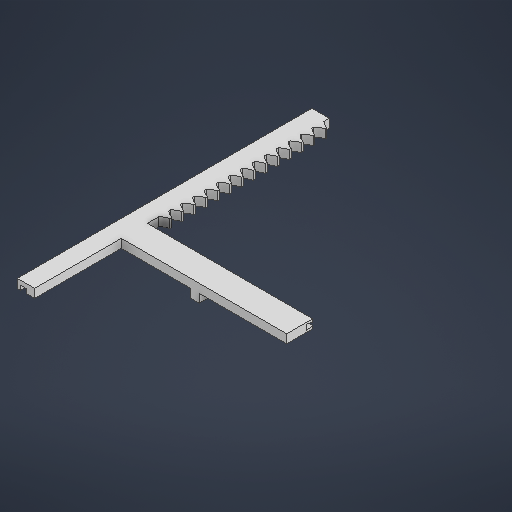
# Autodesk Inventor part: Rack
Saved by Autodesk Inventor 2026.1 (Build 301233020, 233B)
## iProperties
Created: 2025-10-17
Part Number: Rack
Material: Generic
Document SubType Name: Modeling
Designer: alexj
Density: 1 g/cm^3
Appearance: Default
Author: alexj
Autodesk Inventor part; units mm, degrees
ref_plane "YZ Plane" through (0, 0, 0) normal (1, 0, 0) x (0, 1, 0)
ref_plane "XZ Plane" through (0, 0, 0) normal (0, 1, 0) x (-1, 0, 0)
ref_plane "XY Plane" through (0, 0, 0) normal (0, 0, 1) x (1, 0, 0)
sketch "Sketch1" plane through (0, 0, 0) normal (0, 1, 0) x (-1, 0, 0)
  line L0 (0, 0) -> (10, 0)
  line L1 (10, 0) -> (10, -170)
  line L2 (10, -170) -> (0, -170)
  line L3 (0, -170) -> (0, 0)
  dimension "d0" = 170
  dimension "d1" = 10
  constraints: 8 end point, 2 parallel, 1 horizontal, 1 perpendicular
  measures "d0" distance of L0.end L1.end
  measures "d1" distance of L1.end L2.end
extrude "Extrusion1" add sketch "Sketch1" along normal blind 5
sketch "Sketch2" plane through (-10, 0, 0) normal (0, 0, 1) x (1, 0, 0)
  line L0 (2, 0) -> (2, 2.5)
  line L1 (2, 2.5) -> (5, 2.5)
  line L2 (0, 0) -> (0, 5) projected
  line L3 (5, 2.5) -> (5, 0)
  line L4 (0, 0) -> (10, 0) projected
  dimension "d6" = 2
  dimension "d9" = 3
  dimension "d75" = 2.5
  constraints: 6 end point, 1 midpoint, 1 perpendicular, 1 point on line, 1 vertical
  measures "d6" distance between parallel lines of L2 L0
  measures "d9" distance of L0.end L1.end
  measures "d75" distance between parallel lines of L4 L1
sketch "Sketch4" plane through (0, 5, 0) normal (0, 1, 0) x (1, 0, 0)
  line L0 (95.426, 50) -> (95.426, 65)
  line L1 (95.426, 65) -> (0, 65)
  line L2 (95.426, 50) -> (0, 50)
  line L3 (-10, 0) -> (0, 0) projected
  line L4 (0, 0) -> (0, 170) projected
  line L5 (0, 50) -> (0, 65)
  dimension "d107" = 95.426
  dimension "d108" = 15
  dimension "d109" = 50
  constraints: 9 end point, 2 perpendicular, 1 horizontal, 1 parallel, 1 point on line, 1 vertical
  measures "d107" distance from line of L3.end L0
  measures "d108" distance between parallel lines of L1 L2
  measures "d109" distance from line of L3.end L2
extrude "Extrusion4" add sketch "Sketch4" against normal blind 5
sketch "Sketch6" plane through (0, 5, 0) normal (0, 1, 0) x (1, 0, 0)
  line L0 (0, 0) -> (0, 170) projected
  line L1 (95.426, 50) -> (95.426, 65) projected
  arc A0 (4.0959, 156.5581) -> (0, 154.1943) centre (6.5788, 147.5251) ccw
  arc A1 (4.0959, 157.6362) -> (4.0959, 156.5581) centre (9.5694, 157.0972) ccw
  arc A2 (0, 160) -> (4.0959, 157.6362) centre (6.5788, 166.6692) ccw
  line L2 (0, 154.1943) -> (0, 160)
  arc A3 (4.0959, 163.4421) -> (0, 161.0783) centre (6.5788, 154.4091) ccw
  arc A4 (4.0959, 164.5202) -> (4.0959, 163.4421) centre (9.5694, 163.9812) ccw
  arc A5 (0, 166.884) -> (4.0959, 164.5202) centre (6.5788, 173.5532) ccw
  arc A6 (4.0959, 149.6741) -> (0, 147.3103) centre (6.5788, 140.6411) ccw
  arc A7 (4.0959, 150.7522) -> (4.0959, 149.6741) centre (9.5694, 150.2132) ccw
  arc A8 (0, 153.116) -> (4.0959, 150.7522) centre (6.5788, 159.7852) ccw
  arc A9 (4.0959, 142.7901) -> (0, 140.4263) centre (6.5788, 133.7571) ccw
  arc A10 (4.0959, 143.8682) -> (4.0959, 142.7901) centre (9.5694, 143.3292) ccw
  arc A11 (0, 146.232) -> (4.0959, 143.8682) centre (6.5788, 152.9012) ccw
  arc A12 (4.0959, 135.9061) -> (0, 133.5423) centre (6.5788, 126.8731) ccw
  arc A13 (4.0959, 136.9842) -> (4.0959, 135.9061) centre (9.5694, 136.4452) ccw
  arc A14 (0, 139.348) -> (4.0959, 136.9842) centre (6.5788, 146.0172) ccw
  arc A15 (4.0959, 129.0221) -> (0, 126.6583) centre (6.5788, 119.9891) ccw
  arc A16 (4.0959, 130.1002) -> (4.0959, 129.0221) centre (9.5694, 129.5612) ccw
  arc A17 (0, 132.464) -> (4.0959, 130.1002) centre (6.5788, 139.1332) ccw
  arc A18 (4.0959, 122.1381) -> (0, 119.7743) centre (6.5788, 113.1051) ccw
  arc A19 (4.0959, 123.2162) -> (4.0959, 122.1381) centre (9.5694, 122.6772) ccw
  arc A20 (0, 125.58) -> (4.0959, 123.2162) centre (6.5788, 132.2492) ccw
  arc A21 (4.0959, 115.2541) -> (0, 112.8903) centre (6.5788, 106.2211) ccw
  arc A22 (4.0959, 116.3322) -> (4.0959, 115.2541) centre (9.5694, 115.7932) ccw
  arc A23 (0, 118.696) -> (4.0959, 116.3322) centre (6.5788, 125.3652) ccw
  arc A24 (4.0959, 108.3701) -> (0, 106.0063) centre (6.5788, 99.3371) ccw
  arc A25 (4.0959, 109.4482) -> (4.0959, 108.3701) centre (9.5694, 108.9092) ccw
  arc A26 (0, 111.812) -> (4.0959, 109.4482) centre (6.5788, 118.4812) ccw
  arc A27 (4.0959, 101.4861) -> (0, 99.1223) centre (6.5788, 92.4531) ccw
  arc A28 (4.0959, 102.5642) -> (4.0959, 101.4861) centre (9.5694, 102.0252) ccw
  arc A29 (0, 104.928) -> (4.0959, 102.5642) centre (6.5788, 111.5972) ccw
  arc A30 (4.0959, 94.6021) -> (0, 92.2383) centre (6.5788, 85.5691) ccw
  arc A31 (4.0959, 95.6802) -> (4.0959, 94.6021) centre (9.5694, 95.1412) ccw
  arc A32 (0, 98.044) -> (4.0959, 95.6802) centre (6.5788, 104.7132) ccw
  arc A33 (4.0959, 87.7181) -> (0, 85.3543) centre (6.5788, 78.6851) ccw
  arc A34 (4.0959, 88.7962) -> (4.0959, 87.7181) centre (9.5694, 88.2572) ccw
  arc A35 (0, 91.16) -> (4.0959, 88.7962) centre (6.5788, 97.8292) ccw
  arc A36 (4.0959, 80.8341) -> (0, 78.4703) centre (6.5788, 71.8011) ccw
  arc A37 (4.0959, 81.9122) -> (4.0959, 80.8341) centre (9.5694, 81.3732) ccw
  arc A38 (0, 84.276) -> (4.0959, 81.9122) centre (6.5788, 90.9452) ccw
  arc A39 (4.0959, 73.9501) -> (0, 71.5863) centre (6.5788, 64.9171) ccw
  arc A40 (4.0959, 75.0282) -> (4.0959, 73.9501) centre (9.5694, 74.4892) ccw
  arc A41 (0, 77.392) -> (4.0959, 75.0282) centre (6.5788, 84.0612) ccw
  point P0 (0, 65)
  point P1 (0, 154.1943)
  point P2 (0, 166.884)
  point P3 (0, 161.0783)
  point P4 (0, 77.392)
  point P5 (0, 71.5863)
  point P6 (0, 84.276)
  point P7 (0, 78.4703)
  point P8 (0, 91.16)
  point P9 (0, 85.3543)
  point P10 (0, 98.044)
  point P11 (0, 92.2383)
  point P12 (0, 104.928)
  point P13 (0, 99.1223)
  point P14 (0, 111.812)
  point P15 (0, 106.0063)
  point P16 (0, 118.696)
  point P17 (0, 112.8903)
  point P18 (0, 125.58)
  point P19 (0, 119.7743)
  point P20 (0, 132.464)
  point P21 (0, 126.6583)
  point P22 (0, 139.348)
  point P23 (0, 133.5423)
  point P24 (0, 146.232)
  point P25 (0, 140.4263)
  point P26 (0, 153.116)
  point P27 (0, 147.3103)
  dimension "d80" = 6.884
  dimension "d88" = 6.884
  dimension "d200" = 5.5
  dimension "d201" = 9.368
  dimension "d202" = 95.426
  dimension "d203" = 95.426
  dimension "d204" = 85.8566
  dimension "d205" = 88.8472
  dimension "d206" = 88.8472
  dimension "d207" = 91.3301
  dimension "d208" = 91.3301
  dimension "d209" = 95.426
  dimension "d210" = 95.426
  dimension "d211" = 95.426
  dimension "d212" = 95.426
  dimension "d213" = 95.426
  dimension "d214" = 95.426
  dimension "d215" = 95.426
  dimension "d216" = 95.426
  dimension "d217" = 95.426
  dimension "d218" = 95.426
  dimension "d219" = 95.426
  dimension "d220" = 95.426
  dimension "d221" = 95.426
  dimension "d222" = 95.426
  dimension "d223" = 95.426
  dimension "d224" = 95.426
  dimension "d225" = 95.426
  dimension "d226" = 95.426
  dimension "d227" = 95.426
  dimension "d228" = 95.426
  dimension "d229" = 95.426
  dimension "d230" = 95.426
  dimension "d231" = 95.426
  dimension "d232" = 95.426
  dimension "d233" = 95.426
  dimension "d234" = 95.426
  dimension "d235" = 95.426
  dimension "d236" = 95.426
  dimension "d237" = 131.0291
  dimension "d238" = 139.594
  dimension "d239" = 135.4148
  dimension "d240" = 134.6518
  dimension "d241" = 130.6206
  dimension "d242" = 129.8867
  dimension "d243" = 126.0203
  dimension "d244" = 125.3186
  dimension "d245" = 121.6357
  dimension "d246" = 120.97
  dimension "d247" = 117.4912
  dimension "d248" = 116.8654
  dimension "d249" = 113.6128
  dimension "d250" = 113.0312
  dimension "d251" = 110.0288
  dimension "d252" = 109.496
  dimension "d253" = 106.7689
  dimension "d254" = 106.2896
  dimension "d255" = 103.8636
  dimension "d256" = 103.4426
  dimension "d257" = 101.3432
  dimension "d258" = 100.9853
  dimension "d259" = 99.2373
  dimension "d260" = 98.9468
  dimension "d261" = 97.5726
  constraints: 91 vertical alignment, 84 point on circle, 42 centre point, 40 equal radius, 2 end point, 1 other
  measures "d80" distance of A0.start A3.start
  measures "d88" distance of A0.start A6.start
  measures "d200" radius of A4
  measures "d201" radius of A5
  measures "d202" distance from line of L1.end L2
  measures "d203" distance from line of L1.start L2
  measures "d204" distance from line of A4.centre L1
  measures "d205" distance from line of A5.centre L1
  measures "d206" distance from line of A3.centre L1
  measures "d207" distance from line of A4.start L1
  measures "d208" distance from line of A3.start L1
  measures "d209" distance from line of point (0, 166.884) L1
  measures "d210" distance from line of point (0, 161.078) L1
  measures "d211" distance from line of point (0, 160) L1
  measures "d212" distance from line of point (0, 154.194) L1
  measures "d213" distance from line of point (0, 153.116) L1
  measures "d214" distance from line of point (0, 147.31) L1
  measures "d215" distance from line of point (0, 146.232) L1
  measures "d216" distance from line of point (0, 140.426) L1
  measures "d217" distance from line of point (0, 139.348) L1
  measures "d218" distance from line of point (0, 133.542) L1
  measures "d219" distance from line of point (0, 132.464) L1
  measures "d220" distance from line of point (0, 126.658) L1
  measures "d221" distance from line of point (0, 125.58) L1
  measures "d222" distance from line of point (0, 119.774) L1
  measures "d223" distance from line of point (0, 118.696) L1
  measures "d224" distance from line of point (0, 112.89) L1
  measures "d225" distance from line of point (0, 111.812) L1
  measures "d226" distance from line of point (0, 106.006) L1
  measures "d227" distance from line of point (0, 104.928) L1
  measures "d228" distance from line of point (0, 99.122) L1
  measures "d229" distance from line of point (0, 98.044) L1
  measures "d230" distance from line of point (0, 92.238) L1
  measures "d231" distance from line of point (0, 91.16) L1
  measures "d232" distance from line of point (0, 85.354) L1
  measures "d233" distance from line of point (0, 84.276) L1
  measures "d234" distance from line of point (0, 78.47) L1
  measures "d235" distance from line of point (0, 77.392) L1
  measures "d236" distance from line of point (0, 71.586) L1
  measures "d237" distance of L1.end A4.centre
  measures "d238" distance of L1.end point (0, 166.884)
  measures "d239" distance of L1.end point (0, 161.078)
  measures "d240" distance of L1.end point (0, 160)
  measures "d241" distance of L1.end point (0, 154.194)
  measures "d242" distance of L1.end point (0, 153.116)
  measures "d243" distance of L1.end point (0, 147.31)
  measures "d244" distance of L1.end point (0, 146.232)
  measures "d245" distance of L1.end point (0, 140.426)
  measures "d246" distance of L1.end point (0, 139.348)
  measures "d247" distance of L1.end point (0, 133.542)
  measures "d248" distance of L1.end point (0, 132.464)
  measures "d249" distance of L1.end point (0, 126.658)
  measures "d250" distance of L1.end point (0, 125.58)
  measures "d251" distance of L1.end point (0, 119.774)
  measures "d252" distance of L1.end point (0, 118.696)
  measures "d253" distance of L1.end point (0, 112.89)
  measures "d254" distance of L1.end point (0, 111.812)
  measures "d255" distance of L1.end point (0, 106.006)
  measures "d256" distance of L1.end point (0, 104.928)
  measures "d257" distance of L1.end point (0, 99.122)
  measures "d258" distance of L1.end point (0, 98.044)
  measures "d259" distance of L1.end point (0, 92.238)
  measures "d260" distance of L1.end point (0, 91.16)
  measures "d261" distance of L1.end point (0, 85.354)
extrude "Extrusion6" add sketch "Sketch6" against normal blind 5
extrude "Extrusion10" cut sketch "Sketch2" against normal blind 300
sketch "Sketch9" plane through (0, 0, 0) normal (0, -1, 0) x (1, 0, 0)
  line L0 (95.426, -65) -> (0, -65) projected
  line L1 (40, -50) -> (45, -50)
  line L2 (45, -50) -> (45, -65)
  line L3 (45, -65) -> (40, -65)
  line L4 (40, -65) -> (40, -50)
  line L5 (95.426, -50) -> (0, -50) projected
  line L6 (-10, -170) -> (-10, 0) projected
  point P0 (0, 0)
  dimension "d93" = 5
  dimension "d94" = 55
  constraints: 8 end point, 2 parallel, 2 point on line, 1 horizontal, 1 perpendicular
  measures "d93" distance between parallel lines of L2 L4
  measures "d94" distance between parallel lines of L6 L2
extrude "Extrusion11" add sketch "Sketch9" along normal blind 4.95
chamfer "Chamfer1" distance 4.75 angle 45 1 edges at (42.5, -4.95, -65)
sketch "Sketch11" plane through (95.426, 5, -50) normal (1, 0, 0) x (0, 0, -1)
  line L0 (15, 0) -> (15, -5) projected
  line L1 (11.5, -1) -> (11.5, -4)
  line L2 (11.5, -4) -> (15, -3.3829)
  line L3 (11.5, -1) -> (15, -1.6171)
  point P0 (11.5, -2.5)
  point P1 (15, -2.5)
  dimension "d100" = 3.5
  dimension "d101" = 80
  dimension "d104" = 3
  constraints: 6 end point, 2 midpoint, 2 point on line, 1 equal length, 1 horizontal alignment, 1 vertical
  measures "d100" distance between parallel lines of L0 L1
  measures "d101" angle of L3 L1
  measures "d104" distance of L1.start L1.end
extrude "Extrusion12" cut sketch "Sketch11" against normal blind 45
body "Solid1"
